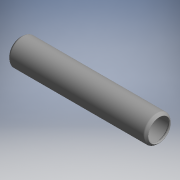
# Autodesk Inventor part: 007R-1.8150
Saved by Autodesk Inventor 2017.3 (Build 213256000, 256)
## iProperties
Part Number: 007R-1.8150
Material: Generic
Catalog Web Link: www.cadenas.de
Description: Tube-Original Line - Standard Air Cylinders
Vendor: BIMBA
Document SubType Name: Modeling
Designer: partserver
Manufacturer: BIMBA
Mass: 0.613427 g
Surface Area: 25.8111 cm^2
Volume: 0.613427 cm^3
Density: 1 g/cm^3
Appearance: PSOLRGB-180-180-180
Category: PARTsolutions
Company: BIMBA
Title: 007R-1.8150
Author: Cadenas PARTsolutions
Comments: Original Line - Standard Air Cylinders
PSOL_IDENT_0: {$CADENAS_DATA\23d-libs\bimba\bimba_brand\bimba_imperial\bimba_full_line\original_line_cylinders\sta
PSOL_IDENT_1: ndard_air_cylinders\tube.prj},201 {VTYP=3D},{NB=007R-1.8150},{LINA=007R-1.8150},{NN=Tube},{DATE=19.0
PSOL_IDENT_2: 1.2022 10:19:38},{GEOMDATE=03.03.2020 12:52:40},{VERSION=},{LINEID=10},{WBVAR=MNT,ACTING,NR,L,FOURHO
PSOL_IDENT_3: LES,SR,K},{WBNUMERIC=L,FOURHOLES}  {NB=007R-1.8150},{LINA=007R-1.8150},{KT=DUMMY},{PN=007R-1.8150},{
PSOL_IDENT_4: BORE=0.31250000},{BOREPN=007},{MNT=},{MNTALG='' , 'Front Nose' , 'BF' , 'Front Block'},{ACTING=R},{A
PSOL_IDENT_5: CTINGALG= '' , 'Single Acting' , 'R' , 'Reverse/Double Acting' },{NR=},{NRALG= '' , 'N/A' },{L=1.815
PSOL_IDENT_6: 0},{OD=0.3590},{ODN=0.3590},{ODP=0.6050},{ODB=0.0000},{ID=0.3215},{DV=0.09400000},{LV=0.37500000},{L
PSOL_IDENT_7: V1=0.03000000},{G=0.0220},{FOURHOLES=0},{AA=0.3250},{BB=0.0620},{SR=},{SRALG= 'C' , 'Carbon Steel Ro
PSOL_IDENT_8: d' , 'SR' , '303 Stainless Steel Rod' , '' , '303 Stainless Steel Rod'},{KALG= '', 'Standard' , 'K'
PSOL_IDENT_9: , 'Ports Rotated 90deg' },{K=}
NB: 007R-1.8150
NN: Tube
NT: Original Line - Standard Air Cylinders
NBSYN: $PN.
LINA: 007R-1.8150
CATALOG: Bimba Products
BORE: 0
BOREPN: 007
MNT: Front Nose
MNTALG: '' , 'Front Nose' , 'BF' , 'Front Block'
ACTING: Reverse/Double Acting
NR: N/A
L: 1.815
ODN: 0.359
ODP: 0.605
ODB: 0
ID: 0.3215
DV: 0.094
LV: 0.375
LV1: 0.03
G: 0.022
FOURHOLES: 0
AA: 0.325
BB: 0.062
SR: 303 Stainless Steel Rod
K: Standard
SUPPLIER: BIMBA
ARTICLENO: 007R-1.8150
BOMINFO: 007R-1.8150
CREATOR: CADENAS GmbH
Autodesk Inventor part; units mm, degrees
sketch "Sketch_1" plane through (0, 0, 0) normal (0, 0, 1) x (1, 0, 0)
  line L0 (46.101, 0) -> (0, 0)
  arc A0 (-0.445, 3.8695) -> (-0.445, 3.6899) centre (-0.3552, 3.7797) ccw
  line L1 (-0.445, 3.6899) -> (-0.2794, 3.5243)
  line L2 (-0.2794, 3.5243) -> (0, 3.5243)
  line L3 (0, 3.5243) -> (0.5588, 4.0831)
  line L4 (0.5588, 4.0831) -> (45.5422, 4.0831)
  line L5 (45.5422, 4.0831) -> (46.101, 3.5243)
  line L6 (46.101, 3.5243) -> (46.3804, 3.5243)
  line L7 (46.3804, 3.5243) -> (46.546, 3.6899)
  arc A1 (46.546, 3.6899) -> (46.546, 3.8695) centre (46.4562, 3.7797) ccw
  line L8 (46.546, 3.8695) -> (46.0199, 4.3956)
  arc A2 (46.0199, 4.3956) -> (45.6247, 4.5593) centre (45.6247, 4.0005) ccw
  line L9 (45.6247, 4.5593) -> (0.4763, 4.5593)
  arc A3 (0.4763, 4.5593) -> (0.0811, 4.3956) centre (0.4762, 4.0005) ccw
  line L10 (0.0811, 4.3956) -> (-0.445, 3.8695)
  constraints: 22 end point, 8 point on circle, 4 centre point
revolve "Revolution1" add sketch "Sketch_1" angle 360 about axis through (46.101, 0, 0) along (1, 0, 0)
ref_plane "cp1_XY" through (23.0505, 0, 4.5593) normal (1, 0, 0) x (0, 0, -1)
ref_plane "cp1_YZ" through (23.0505, 0, 4.5593) normal (0, 0, -1) x (0, 1, 0)
ref_plane "cp1_ZX" through (23.0505, 0, 4.5593) normal (0, 1, 0) x (1, 0, 0)
ref_plane "cp2_XY" through (23.0505, 4.5593, 0) normal (1, 0, 0) x (0, 0, -1)
ref_plane "cp2_YZ" through (23.0505, 4.5593, 0) normal (0, 0, -1) x (0, 1, 0)
ref_plane "cp2_ZX" through (23.0505, 4.5593, 0) normal (0, 1, 0) x (1, 0, 0)
ref_plane "cp3_XY" through (23.0505, 0, -4.5593) normal (1, 0, 0) x (0, 0, -1)
ref_plane "cp3_YZ" through (23.0505, 0, -4.5593) normal (0, 0, -1) x (0, 1, 0)
ref_plane "cp3_ZX" through (23.0505, 0, -4.5593) normal (0, 1, 0) x (1, 0, 0)
ref_plane "cp4_XY" through (23.0505, -4.5593, 0) normal (1, 0, 0) x (0, 0, -1)
ref_plane "cp4_YZ" through (23.0505, -4.5593, 0) normal (0, 0, -1) x (0, 1, 0)
ref_plane "cp4_ZX" through (23.0505, -4.5593, 0) normal (0, 1, 0) x (1, 0, 0)
ref_plane "tube_front_XY" through (0, 0, 0) normal (1, 0, 0) x (0, 0, -1)
ref_plane "tube_front_YZ" through (0, 0, 0) normal (0, 0, -1) x (0, 1, 0)
ref_plane "tube_front_ZX" through (0, 0, 0) normal (0, 1, 0) x (1, 0, 0)
ref_plane "tube_rear_XY" through (46.101, 0, 0) normal (1, 0, 0) x (0, 0, -1)
ref_plane "tube_rear_YZ" through (46.101, 0, 0) normal (0, 0, -1) x (0, 1, 0)
ref_plane "tube_rear_ZX" through (46.101, 0, 0) normal (0, 1, 0) x (1, 0, 0)
body "Solid1"
